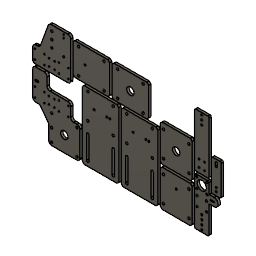
_Sheet Metal Arrangement Model.7c029e5c-e530-4885-910f-0bde3985115b (Autodesk Fusion 360 design; units mm, degrees)
Autodesk Fusion 360 part; units mm, degrees
sketch "Sketch1" plane through (0, 0, 0) normal (0, 0, 1) x (1, 0, 0)
  arc A0 (161.5993, 83.15) -> (155.1993, 83.15) centre (158.3993, 83.15) ccw
  line L0 (250.2493, 11.35) -> (255.2493, 6.35)
  line L1 (321.05, 288.7) -> (230.05, 288.7)
  arc A1 (128.5493, 6.35) -> (136.5493, 14.35) centre (128.5493, 14.35) ccw
  line L2 (161.5993, 83.15) -> (161.5993, 19.55)
  arc A2 (268.9493, 83.15) -> (262.5493, 83.15) centre (265.7493, 83.15) ccw
  line L3 (255.2493, 6.35) -> (346.2493, 6.35)
  line L4 (230.05, 200.7) -> (321.05, 200.7)
  line L5 (142.8993, 11.35) -> (147.8993, 6.35)
  line L6 (262.5493, 19.55) -> (262.5493, 83.15)
  line L7 (225.1993, 19.55) -> (225.1993, 83.15)
  line L8 (6.35, 186.3975) -> (6.35, 216.3975)
  line L9 (455.2118, 103.5874) -> (457.7118, 106.0874)
  arc A3 (56.95, 294.3975) -> (49.4332, 289.1358) centre (56.95, 286.3975) ccw
  line L10 (445.5993, 118.7) -> (445.5993, 209.7)
  line L11 (486.1867, 106.0874) -> (488.6867, 103.5874)
  circle A4 centre (471.9493, 117.85) radius 12.5
  arc A5 (50.7493, 14.35) -> (58.7493, 6.35) centre (58.7493, 14.35) ccw
  circle A6 centre (93.6493, 49.25) radius 10
  circle A7 centre (66.9255, 211.3975) radius 2
  line L12 (117.7, 283.7) -> (117.7, 205.7)
  line L13 (486.2118, 101.1126) -> (483.7118, 103.6126)
  arc A8 (103.35, 178.3975) -> (111.35, 186.3975) centre (103.35, 186.3975) ccw
  line L14 (488.6867, 132.1126) -> (486.1867, 129.6126)
  line L15 (103.35, 178.3975) -> (14.35, 178.3975)
  line L16 (498.2993, 115.95) -> (498.2993, 197.6067)
  arc A9 (6.35, 96.0318) -> (14.35, 88.0318) centre (14.35, 96.0318) ccw
  line L17 (457.7118, 129.6126) -> (455.2118, 132.1126)
  arc A10 (486.2118, 101.1126) -> (488.6867, 103.5874) centre (487.4493, 102.35) ccw
  circle A11 centre (51.9255, 191.3975) radius 2
  circle A12 centre (66.9255, 191.3975) radius 2
  circle A13 centre (471.9493, 117.85) radius 12.5
  arc A14 (457.7118, 129.6126) -> (460.1867, 132.0874) centre (458.9493, 130.85) ccw
  arc A15 (46.35, 164.0475) -> (38.35, 172.0475) centre (38.35, 164.0475) ccw
  line L18 (498.2993, 197.6067) -> (498.2993, 115.95)
  circle A16 centre (12.85, 214.3975) radius 2
  circle A17 centre (104.85, 214.3975) radius 2
  arc A18 (46.35, 164.0475) -> (38.35, 172.0475) centre (38.35, 164.0475) ccw
  circle A19 centre (104.85, 98.0318) radius 2
  line L19 (346.2493, 194.35) -> (351.2493, 189.35)
  arc A20 (111.3468, 126.0475) -> (103.3468, 134.0475) centre (103.3468, 126.0475) ccw
  circle A21 centre (104.85, 124.0318) radius 2
  circle A22 centre (78.85, 98.0318) radius 2
  line L20 (117.7, 283.7) -> (117.7, 205.7)
  circle A23 centre (366.5993, 199.2) radius 3.2
  circle A24 centre (38.8353, 98.0318) radius 2
  circle A25 centre (93.6493, 49.25) radius 10
  circle A26 centre (12.8353, 124.0318) radius 2
  line L21 (326.05, 283.7) -> (321.05, 288.7)
  circle A27 centre (310.55, 279.7) radius 3.2
  arc A28 (6.35, 186.3975) -> (14.35, 178.3975) centre (14.35, 186.3975) ccw
  line L22 (50.7493, 52.1465) -> (50.7493, 14.35)
  line L23 (326.05, 205.7) -> (326.05, 283.7)
  arc A29 (111.3468, 126.0475) -> (103.3468, 134.0475) centre (103.3468, 126.0475) ccw
  arc A30 (111.3468, 100.15) -> (119.3468, 92.15) centre (119.3468, 100.15) ccw
  circle A31 centre (401.5993, 164.2) radius 10
  line L24 (326.05, 283.7) -> (321.05, 288.7)
  arc A32 (103.35, 178.3975) -> (111.35, 186.3975) centre (103.35, 186.3975) ccw
  line L25 (6.35, 164.0475) -> (6.35, 96.0318)
  line L26 (46.35, 142.0475) -> (46.35, 164.0475)
  arc A33 (14.35, 172.0475) -> (6.35, 164.0475) centre (14.35, 164.0475) ccw
  arc A34 (50.7493, 52.1465) -> (49.1493, 56.9465) centre (42.7493, 52.1465) ccw
  line L27 (20.35, 137.5475) -> (15.35, 137.5475)
  circle A35 centre (318.2493, 150.35) radius 2.5
  circle A36 centre (335.7493, 185.35) radius 3.2
  line L28 (454.9493, 144.2) -> (488.9493, 144.2)
  line L29 (491.9493, 245.8549) -> (451.9493, 245.8549)
  circle A37 centre (484.9493, 87.35) radius 2.95
  circle A38 centre (471.9493, 286.0097) radius 2.55
  circle A39 centre (479.4493, 157.2) radius 2.25
  circle A40 centre (471.9493, 274.0097) radius 2.55
  arc A41 (514.3216, 192.5955) -> (509.3216, 192.6178) centre (511.8216, 192.6066) ccw
  arc A42 (495.9493, 96.6) -> (495.9493, 94.1) centre (495.9493, 95.35) ccw
  line L30 (454.9493, 292.0097) -> (488.9493, 292.0097)
  circle A43 centre (458.9493, 61.35) radius 2.75
  arc A44 (505.9493, 84.1) -> (505.9493, 106.6) centre (505.9493, 95.35) ccw
  circle A45 centre (484.9493, 61.35) radius 2.75
  line L31 (522.2993, 200.6067) -> (501.2993, 200.6067)
  line L32 (505.9493, 106.6) -> (491.9493, 106.6)
  circle A46 centre (511.7993, 122.95) radius 2.55
  circle A47 centre (471.9493, 48.35) radius 2.55
  arc A48 (525.2993, 197.6067) -> (522.2993, 200.6067) centre (522.2993, 197.6067) ccw
  line L33 (509.277, 182.6179) -> (509.3216, 192.6178)
  line L34 (491.9493, 192.8549) -> (451.9493, 192.8549)
  arc A49 (488.9493, 144.2) -> (491.9493, 147.2) centre (488.9493, 147.2) ccw
  arc A50 (451.9493, 147.2) -> (454.9493, 144.2) centre (454.9493, 147.2) ccw
  line L35 (498.2993, 146.9567) -> (525.2993, 146.9567)
  arc A51 (491.9493, 134.85) -> (488.9493, 137.85) centre (488.9493, 134.85) ccw
  arc A52 (451.9493, 9.35) -> (454.9493, 6.35) centre (454.9493, 9.35) ccw
  arc A53 (501.2993, 200.6067) -> (498.2993, 197.6067) centre (501.2993, 197.6067) ccw
  line L36 (451.9493, 251.5097) -> (491.9493, 251.5097)
  line L37 (505.9493, 94.1) -> (495.9493, 94.1)
  line L38 (491.9493, 147.2) -> (491.9493, 289.0097)
  arc A54 (491.9493, 134.85) -> (488.9493, 137.85) centre (488.9493, 134.85) ccw
  arc A55 (498.2993, 115.95) -> (501.2993, 112.95) centre (501.2993, 115.95) ccw
  circle A56 centre (471.9493, 36.35) radius 2.55
  line L39 (451.9493, 289.0097) -> (451.9493, 147.2)
  arc A57 (488.9493, 6.35) -> (491.9493, 9.35) centre (488.9493, 9.35) ccw
  line L40 (491.9493, 84.1) -> (505.9493, 84.1)
  line L41 (495.9493, 96.6) -> (505.9493, 96.6)
  line L42 (501.2993, 112.95) -> (522.2993, 112.95)
  line L43 (491.9493, 84.1) -> (505.9493, 84.1)
  arc A58 (522.2993, 112.95) -> (525.2993, 115.95) centre (522.2993, 115.95) ccw
  arc A59 (505.9493, 94.1) -> (505.9493, 96.6) centre (505.9493, 95.35) ccw
  arc A60 (491.9493, 289.0097) -> (488.9493, 292.0097) centre (488.9493, 289.0097) ccw
  line L44 (491.9493, 190.0274) -> (451.9493, 190.0274)
  circle A61 centre (464.4493, 177.2) radius 2.25
  line L45 (491.9493, 147.2) -> (491.9493, 289.0097)
  circle A62 centre (458.9493, 87.35) radius 2.95
  line L46 (505.9493, 106.6) -> (491.9493, 106.6)
  arc A63 (505.9493, 84.1) -> (505.9493, 106.6) centre (505.9493, 95.35) ccw
  line L47 (491.9493, 187.2) -> (451.9493, 187.2)
  line L48 (491.9493, 106.6) -> (491.9493, 134.85)
  arc A64 (498.2993, 115.95) -> (501.2993, 112.95) centre (501.2993, 115.95) ccw
  line L49 (491.9493, 106.6) -> (491.9493, 134.85)
  arc A65 (525.2993, 197.6067) -> (522.2993, 200.6067) centre (522.2993, 197.6067) ccw
  line L50 (491.9493, 9.35) -> (491.9493, 84.1)
  arc A66 (522.2993, 112.95) -> (525.2993, 115.95) centre (522.2993, 115.95) ccw
  line L51 (451.9493, 134.85) -> (451.9493, 9.35)
  line L52 (218.7, 283.7) -> (213.7, 288.7)
  line L53 (243.8993, 189.35) -> (238.8993, 194.35)
  line L54 (230.05, 288.7) -> (225.05, 283.7)
  line L55 (357.5993, 102.35) -> (357.5993, 11.35)
  line L56 (213.7, 200.7) -> (218.7, 205.7)
  circle A67 centre (240.55, 209.7) radius 3.2
  line L57 (218.7, 283.7) -> (213.7, 288.7)
  line L58 (213.7, 288.7) -> (122.7, 288.7)
  line L59 (238.8993, 194.35) -> (147.8993, 194.35)
  circle A68 centre (203.2, 209.7) radius 3.2
  circle A69 centre (275.55, 244.7) radius 10
  circle A70 centre (436.5993, 91.85) radius 3.2
  line L60 (225.05, 205.7) -> (230.05, 200.7)
  line L61 (225.05, 283.7) -> (225.05, 205.7)
  circle A71 centre (240.55, 279.7) radius 3.2
  line L62 (445.5993, 209.7) -> (440.5993, 214.7)
  circle A72 centre (228.3993, 185.35) radius 3.2
  line L63 (445.5993, 102.35) -> (440.5993, 107.35)
  line L64 (440.5993, 6.35) -> (445.5993, 11.35)
  line L65 (122.7, 288.7) -> (117.7, 283.7)
  circle A73 centre (265.7493, 185.35) radius 3.2
  line L66 (117.7, 205.7) -> (122.7, 200.7)
  circle A74 centre (58.8493, 49.25) radius 3
  arc A75 (28.2353, 84.8318) -> (21.8353, 88.0318) centre (21.8353, 80.0318) ccw
  line L67 (28.2353, 84.8318) -> (49.1493, 56.9465)
  arc A76 (460.1867, 103.6126) -> (457.7118, 106.0874) centre (458.9493, 104.85) ccw
  arc A77 (483.7118, 132.0874) -> (486.1867, 129.6126) centre (484.9493, 130.85) ccw
  circle A78 centre (58.8493, 14.45) radius 3
  arc A79 (457.6867, 134.5874) -> (455.2118, 132.1126) centre (456.4493, 133.35) ccw
  line L68 (21.8353, 88.0318) -> (14.35, 88.0318)
  circle A80 centre (12.85, 188.3975) radius 2
  line L69 (111.35, 186.3975) -> (111.35, 286.3975)
  circle A81 centre (51.9255, 211.3975) radius 2
  arc A82 (46.35, 142.0475) -> (54.35, 134.0475) centre (54.35, 142.0475) ccw
  arc A83 (50.7493, 52.1465) -> (49.1493, 56.9465) centre (42.7493, 52.1465) ccw
  circle A84 centre (66.3493, 121.0318) radius 2
  arc A85 (46.35, 142.0475) -> (54.35, 134.0475) centre (54.35, 142.0475) ccw
  line L70 (50.7493, 14.35) -> (50.7493, 52.1465)
  arc A86 (486.1867, 106.0874) -> (483.7118, 103.6126) centre (484.9493, 104.85) ccw
  arc A87 (488.6867, 132.1126) -> (486.2118, 134.5874) centre (487.4493, 133.35) ccw
  line L71 (14.35, 178.3975) -> (103.35, 178.3975)
  circle A88 centre (38.85, 214.3975) radius 2
  circle A89 centre (78.85, 188.3975) radius 2
  line L72 (488.9493, 137.85) -> (454.9493, 137.85)
  line L73 (457.6867, 134.5874) -> (460.1867, 132.0874)
  circle A90 centre (104.85, 188.3975) radius 2
  line L74 (357.5993, 209.7) -> (357.5993, 118.7)
  circle A91 centre (78.85, 214.3975) radius 2
  line L75 (488.9493, 137.85) -> (454.9493, 137.85)
  line L76 (346.2493, 194.35) -> (255.2493, 194.35)
  line L77 (225.05, 205.7) -> (230.05, 200.7)
  line L78 (238.8993, 194.35) -> (243.8993, 189.35)
  line L79 (225.05, 283.7) -> (225.05, 205.7)
  line L80 (218.7, 205.7) -> (218.7, 283.7)
  line L81 (321.05, 288.7) -> (230.05, 288.7)
  line L82 (230.05, 200.7) -> (321.05, 200.7)
  line L83 (362.5993, 113.7) -> (440.5993, 113.7)
  line L84 (213.7, 288.7) -> (122.7, 288.7)
  circle A92 centre (335.7493, 115.35) radius 3.2
  circle A93 centre (203.2, 279.7) radius 3.2
  line L85 (357.5993, 11.35) -> (362.5993, 6.35)
  line L86 (122.7, 200.7) -> (213.7, 200.7)
  line L87 (440.5993, 107.35) -> (362.5993, 107.35)
  line L88 (142.8993, 189.35) -> (147.8993, 194.35)
  line L89 (440.5993, 113.7) -> (445.5993, 118.7)
  arc A94 (332.5493, 19.55) -> (338.9493, 19.55) centre (335.7493, 19.55) ccw
  circle A95 centre (133.2, 209.7) radius 3.2
  line L90 (357.5993, 102.35) -> (357.5993, 11.35)
  circle A96 centre (436.5993, 129.2) radius 3.2
  line L91 (362.5993, 113.7) -> (440.5993, 113.7)
  line L92 (58.7493, 6.35) -> (128.5493, 6.35)
  line L93 (250.2493, 189.35) -> (255.2493, 194.35)
  line L94 (357.5993, 118.7) -> (362.5993, 113.7)
  line L95 (230.05, 288.7) -> (225.05, 283.7)
  circle A97 centre (133.2, 279.7) radius 3.2
  circle A98 centre (366.5993, 91.85) radius 3.2
  line L96 (122.7, 200.7) -> (213.7, 200.7)
  line L97 (255.2493, 194.35) -> (250.2493, 189.35)
  line L98 (445.5993, 209.7) -> (440.5993, 214.7)
  circle A99 centre (275.55, 244.7) radius 10
  line L99 (338.9493, 83.15) -> (338.9493, 19.55)
  line L100 (147.8993, 194.35) -> (142.8993, 189.35)
  line L101 (332.5493, 19.55) -> (332.5493, 83.15)
  line L102 (501.2993, 112.95) -> (522.2993, 112.95)
  line L103 (514.3216, 192.5955) -> (514.2769, 182.5956)
  circle A100 centre (471.9493, 12.35) radius 2.55
  circle A101 centre (511.7993, 132.95) radius 2.55
  line L104 (454.9493, 6.35) -> (488.9493, 6.35)
  circle A102 centre (471.9493, 262.0097) radius 2.55
  circle A103 centre (464.4493, 157.2) radius 2.25
  line L105 (451.9493, 248.6823) -> (491.9493, 248.6823)
  line L106 (488.9493, 292.0097) -> (454.9493, 292.0097)
  line L107 (454.9493, 6.35) -> (488.9493, 6.35)
  circle A104 centre (479.4493, 177.2) radius 2.25
  arc A105 (451.9493, 147.2) -> (454.9493, 144.2) centre (454.9493, 147.2) ccw
  arc A106 (488.9493, 144.2) -> (491.9493, 147.2) centre (488.9493, 147.2) ccw
  arc A107 (451.9493, 9.35) -> (454.9493, 6.35) centre (454.9493, 9.35) ccw
  arc A108 (501.2993, 200.6067) -> (498.2993, 197.6067) centre (501.2993, 197.6067) ccw
  line L108 (491.9493, 9.35) -> (491.9493, 84.1)
  line L109 (525.2993, 143.3658) -> (498.2993, 143.3658)
  arc A109 (509.277, 182.6179) -> (514.2769, 182.5956) centre (511.7769, 182.6067) ccw
  arc A110 (491.9493, 289.0097) -> (488.9493, 292.0097) centre (488.9493, 289.0097) ccw
  arc A111 (488.9493, 6.35) -> (491.9493, 9.35) centre (488.9493, 9.35) ccw
  line L110 (522.2993, 200.6067) -> (501.2993, 200.6067)
  circle A112 centre (471.9493, 24.35) radius 2.55
  line L111 (454.9493, 144.2) -> (488.9493, 144.2)
  arc A113 (454.9493, 292.0097) -> (451.9493, 289.0097) centre (454.9493, 289.0097) ccw
  arc A114 (454.9493, 292.0097) -> (451.9493, 289.0097) centre (454.9493, 289.0097) ccw
  arc A115 (155.1993, 19.55) -> (161.5993, 19.55) centre (158.3993, 19.55) ccw
  line L112 (147.8993, 6.35) -> (238.8993, 6.35)
  line L113 (268.9493, 83.15) -> (268.9493, 19.55)
  circle A116 centre (283.2493, 150.35) radius 2.5
  circle A117 centre (265.7493, 115.35) radius 3.2
  line L114 (147.8993, 6.35) -> (238.8993, 6.35)
  arc A118 (136.5493, 84.15) -> (128.5493, 92.15) centre (128.5493, 84.15) ccw
  circle A119 centre (210.8993, 150.35) radius 2.5
  circle A120 centre (128.4493, 14.45) radius 3
  line L115 (255.2493, 6.35) -> (346.2493, 6.35)
  arc A121 (128.5493, 6.35) -> (136.5493, 14.35) centre (128.5493, 14.35) ccw
  circle A122 centre (175.8993, 150.35) radius 2.5
  circle A123 centre (158.3993, 115.35) radius 3.2
  line L116 (243.8993, 11.35) -> (238.8993, 6.35)
  arc A124 (262.5493, 19.55) -> (268.9493, 19.55) centre (265.7493, 19.55) ccw
  circle A125 centre (228.3993, 115.35) radius 3.2
  line L117 (250.2493, 189.35) -> (250.2493, 11.35)
  line L118 (440.5993, 107.35) -> (362.5993, 107.35)
  line L119 (351.2493, 189.35) -> (346.2493, 194.35)
  line L120 (54.35, 134.0475) -> (103.3468, 134.0475)
  line L121 (58.7493, 6.35) -> (128.5493, 6.35)
  line L122 (250.2493, 189.35) -> (250.2493, 11.35)
  circle A126 centre (436.5993, 21.85) radius 3.2
  line L123 (346.2493, 6.35) -> (351.2493, 11.35)
  circle A127 centre (150.7, 244.7) radius 2.5
  line L124 (362.5993, 107.35) -> (357.5993, 102.35)
  line L125 (218.7, 205.7) -> (218.7, 283.7)
  line L126 (119.3468, 92.15) -> (128.5493, 92.15)
  circle A128 centre (366.5993, 129.2) radius 3.2
  line L127 (243.8993, 11.35) -> (243.8993, 189.35)
  arc A129 (338.9493, 83.15) -> (332.5493, 83.15) centre (335.7493, 83.15) ccw
  arc A130 (111.3468, 100.15) -> (119.3468, 92.15) centre (119.3468, 100.15) ccw
  line L128 (440.5993, 214.7) -> (362.5993, 214.7)
  circle A131 centre (66.3493, 101.0318) radius 2
  circle A132 centre (401.5993, 74.35) radius 2.5
  line L129 (128.5493, 92.15) -> (119.3468, 92.15)
  line L130 (357.5993, 11.35) -> (362.5993, 6.35)
  circle A133 centre (366.5993, 21.85) radius 3.2
  line L131 (445.5993, 102.35) -> (440.5993, 107.35)
  line L132 (321.05, 200.7) -> (326.05, 205.7)
  line L133 (111.3468, 100.15) -> (111.3468, 126.0475)
  line L134 (362.5993, 107.35) -> (357.5993, 102.35)
  line L135 (117.7, 205.7) -> (122.7, 200.7)
  line L136 (15.35, 142.5475) -> (20.35, 142.5475)
  circle A134 centre (401.5993, 164.2) radius 10
  line L137 (142.8993, 189.35) -> (142.8993, 11.35)
  line L138 (238.8993, 194.35) -> (147.8993, 194.35)
  line L139 (362.5993, 6.35) -> (440.5993, 6.35)
  line L140 (122.7, 288.7) -> (117.7, 283.7)
  circle A135 centre (158.3993, 185.35) radius 3.2
  line L141 (213.7, 200.7) -> (218.7, 205.7)
  line L142 (362.5993, 6.35) -> (440.5993, 6.35)
  line L143 (440.5993, 113.7) -> (445.5993, 118.7)
  circle A136 centre (51.3493, 101.0318) radius 2
  line L144 (326.05, 205.7) -> (326.05, 283.7)
  line L145 (111.35, 186.3975) -> (111.35, 286.3975)
  line L146 (6.35, 96.0318) -> (6.35, 164.0475)
  circle A137 centre (310.55, 209.7) radius 3.2
  line L147 (440.5993, 6.35) -> (445.5993, 11.35)
  line L148 (243.8993, 11.35) -> (243.8993, 189.35)
  line L149 (362.5993, 214.7) -> (357.5993, 209.7)
  line L150 (357.5993, 118.7) -> (362.5993, 113.7)
  circle A138 centre (78.85, 124.0318) radius 2
  line L151 (351.2493, 11.35) -> (346.2493, 6.35)
  line L152 (142.8993, 189.35) -> (142.8993, 11.35)
  line L153 (440.5993, 214.7) -> (362.5993, 214.7)
  arc A139 (20.35, 137.5475) -> (20.35, 142.5475) centre (20.35, 140.0475) ccw
  line L154 (362.5993, 214.7) -> (357.5993, 209.7)
  line L155 (111.3468, 126.0475) -> (111.3468, 100.15)
  arc A140 (15.35, 142.5475) -> (15.35, 137.5475) centre (15.35, 140.0475) ccw
  line L156 (321.05, 200.7) -> (326.05, 205.7)
  arc A141 (136.5493, 84.15) -> (128.5493, 92.15) centre (128.5493, 84.15) ccw
  arc A142 (225.1993, 19.55) -> (231.5993, 19.55) centre (228.3993, 19.55) ccw
  line L157 (136.5493, 14.35) -> (136.5493, 84.15)
  line L158 (147.8993, 6.35) -> (142.8993, 11.35)
  circle A143 centre (218.8993, 150.35) radius 2.5
  line L159 (155.1993, 19.55) -> (155.1993, 83.15)
  line L160 (346.2493, 194.35) -> (255.2493, 194.35)
  line L161 (255.2493, 6.35) -> (250.2493, 11.35)
  circle A144 centre (128.4493, 84.05) radius 3
  line L162 (231.5993, 83.15) -> (231.5993, 19.55)
  line L163 (238.8993, 6.35) -> (243.8993, 11.35)
  line L164 (525.2993, 139.775) -> (498.2993, 139.775)
  line L165 (14.35, 224.3975) -> (20.25, 224.3975)
  line L166 (451.9493, 289.0097) -> (451.9493, 147.2)
  arc A145 (14.35, 224.3975) -> (6.35, 216.3975) centre (14.35, 216.3975) ccw
  line L167 (56.95, 294.3975) -> (103.35, 294.3975)
  line L168 (525.2993, 115.95) -> (525.2993, 197.6067)
  circle A146 centre (59.4255, 259.3975) radius 3
  line L169 (20.25, 224.3975) -> (14.35, 224.3975)
  arc A147 (111.35, 286.3975) -> (103.35, 294.3975) centre (103.35, 286.3975) ccw
  line L170 (445.5993, 118.7) -> (445.5993, 209.7)
  circle A148 centre (59.4255, 239.3975) radius 3
  circle A149 centre (91.9168, 234.3975) radius 2.5
  arc A150 (56.95, 294.3975) -> (49.4332, 289.1358) centre (56.95, 286.3975) ccw
  line L171 (49.4332, 289.1358) -> (27.7668, 229.6593)
  arc A151 (20.25, 224.3975) -> (27.7668, 229.6593) centre (20.25, 232.3975) ccw
  circle A152 centre (59.4255, 279.3975) radius 3
  circle A153 centre (91.9168, 279.3975) radius 2
  line L172 (27.7668, 229.6593) -> (49.4332, 289.1358)
  line L173 (451.9493, 134.85) -> (451.9493, 9.35)
  circle A154 centre (91.9168, 287.3975) radius 2
  arc A155 (14.35, 224.3975) -> (6.35, 216.3975) centre (14.35, 216.3975) ccw
  arc A156 (111.35, 286.3975) -> (103.35, 294.3975) centre (103.35, 286.3975) ccw
  arc A157 (20.25, 224.3975) -> (27.7668, 229.6593) centre (20.25, 232.3975) ccw
  line L174 (445.5993, 11.35) -> (445.5993, 102.35)
  line L175 (445.5993, 11.35) -> (445.5993, 102.35)
  line L176 (103.35, 294.3975) -> (56.95, 294.3975)
  line L177 (525.2993, 197.6067) -> (525.2993, 115.95)
  circle A158 centre (12.8353, 98.0318) radius 2
  line L178 (460.1867, 103.6126) -> (457.6867, 101.1126)
  arc A159 (454.9493, 137.85) -> (451.9493, 134.85) centre (454.9493, 134.85) ccw
  circle A160 centre (58.8493, 84.05) radius 3
  arc A161 (6.35, 186.3975) -> (14.35, 178.3975) centre (14.35, 186.3975) ccw
  circle A162 centre (436.5993, 199.2) radius 3.2
  line L179 (483.7118, 132.0874) -> (486.2118, 134.5874)
  line L180 (351.2493, 11.35) -> (351.2493, 189.35)
  line L181 (14.35, 172.0475) -> (38.35, 172.0475)
  circle A163 centre (51.3493, 121.0318) radius 2
  arc A164 (454.9493, 137.85) -> (451.9493, 134.85) centre (454.9493, 134.85) ccw
  circle A165 centre (38.85, 188.3975) radius 2
  circle A166 centre (38.8353, 124.0318) radius 2
  arc A167 (14.35, 172.0475) -> (6.35, 164.0475) centre (14.35, 164.0475) ccw
  arc A168 (455.2118, 103.5874) -> (457.6867, 101.1126) centre (456.4493, 102.35) ccw
  line L182 (6.35, 216.3975) -> (6.35, 186.3975)
  line L183 (46.35, 164.0475) -> (46.35, 142.0475)
  circle A169 centre (326.2493, 150.35) radius 2.5
  line L184 (38.35, 172.0475) -> (14.35, 172.0475)
  line L185 (351.2493, 11.35) -> (351.2493, 189.35)
  line L186 (357.5993, 209.7) -> (357.5993, 118.7)
  arc A170 (6.35, 96.0318) -> (14.35, 88.0318) centre (14.35, 96.0318) ccw
  line L187 (103.3468, 134.0475) -> (54.35, 134.0475)
  line L188 (14.35, 88.0318) -> (21.8353, 88.0318)
  arc A171 (28.2353, 84.8318) -> (21.8353, 88.0318) centre (21.8353, 80.0318) ccw
  line L189 (28.2353, 84.8318) -> (49.1493, 56.9465)
  arc A172 (50.7493, 14.35) -> (58.7493, 6.35) centre (58.7493, 14.35) ccw
  line L190 (136.5493, 84.15) -> (136.5493, 14.35)
  arc A173 (231.5993, 83.15) -> (225.1993, 83.15) centre (228.3993, 83.15) ccw
extrude "Extrude1" add sketch "Sketch1" along normal blind 6.35 makes body 1 at (459.5277, 34.9667, 0) makes body 2 at (182.7993, 61.95, 0) makes body 3 at (81.5941, 257.7147, 0) makes body 4 at (290.1493, 61.95, 0) makes body 5 at (401.6615, 39.4446, 0) makes body 6 at (461.3971, 242.7935, 0) makes body 7 at (120.6277, 49.25, 0) makes body 8 at (185.754, 244.7, 0) makes body 9 at (248.4086, 244.7, 0) makes body 10 at (428.7407, 164.2, 0) makes body 11 at (521.5651, 149.2044, 0)
equation "d1 = ( 25.4 / 8 ) * 1 mm"
equation "d2 = ( 25.4 / 8 ) * 1 mm"
equation "d3 = ( 25.4 / 8 ) * 1 mm"
equation "d4 = ( 25.4 / 8 ) * 1 mm"
equation "d5 = ( 25.4 / 8 ) * 1 mm"
equation "d8 = ( 25.4 / 8 ) * 1 mm"
